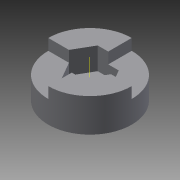
# Autodesk Inventor part: Coil Coupling_1
Saved by Autodesk Inventor 2013 (Build 170138000, 138)
## iProperties
Created: 2013-01-16
Part Number: Coil Coupling_1
Material: Generic
Document SubType Name: Modeling
Designer: Nico
Density: 1 g/cm^3
Author: Nico
Autodesk Inventor part; units mm, degrees
ref_plane "YZ Plane" through (0, 0, 0) normal (1, 0, 0) x (0, 1, 0)
ref_plane "XZ Plane" through (0, 0, 0) normal (0, 1, 0) x (-1, 0, 0)
ref_plane "XY Plane" through (0, 0, 0) normal (0, 0, 1) x (1, 0, 0)
sketch "Sketch1" plane through (0, 0, 0) normal (0, 0, 1) x (1, 0, 0)
  circle A0 centre (0, 0) radius 15
  dimension "d0" = 30
  constraints: 1 centre point, 1 coincident
  measures "d0" diameter of A0
extrude "Extrusion1" add sketch "Sketch1" along normal blind 8
sketch "Sketch2" plane through (0, 0, 8) normal (0, 0, 1) x (1, 0, 0)
  circle A0 centre (0, 0) radius 15 projected
  line L0 (-3.7816, 6.55) -> (0, 6.55)
  line L1 (3.7816, 6.55) -> (7.5633, 0)
  line L2 (7.5633, 0) -> (3.7816, -6.55)
  line L3 (3.7816, -6.55) -> (-3.7816, -6.55)
  line L4 (-3.7816, -6.55) -> (-7.5633, 0)
  line L5 (-7.5633, 0) -> (-3.7816, 6.55)
  line L6 (0, -15) -> (0, -6.55)
  line L7 (-15, 0) -> (-7.5633, 0)
  line L8 (0, 6.55) -> (0, 15)
  line L9 (7.5633, 0) -> (15, 0)
  line L10 (0, 6.55) -> (3.7816, 6.55)
  dimension "d4" = 13.1
  constraints: 22 end point, 6 perpendicular, 4 point on circle, 1 coincident, 1 midpoint, 13 other
  measures "d4" distance between parallel lines of L3 L0
extrude "Extrusion2" add sketch "Sketch2" along normal blind 4 contours A0 L6 L3 L2 L9 | L8 L0 L5 L7 A0
sketch "Sketch3" plane through (0, 0, 8) normal (0, 0, 1) x (1, 0, 0)
  arc A0 (-15, 0) -> (0, -15) centre (0, 0) ccw projected
  line L0 (-3.7816, 6.55) -> (3.7816, 6.55)
  line L1 (3.7816, 6.55) -> (7.5633, 0)
  line L2 (7.5633, 0) -> (3.7816, -6.55)
  line L3 (3.7816, -6.55) -> (-3.7816, -6.55)
  line L4 (-3.7816, -6.55) -> (-7.5633, 0)
  line L5 (-7.5633, 0) -> (-3.7816, 6.55)
  constraints: 12 end point, 1 coincident, 13 other
extrude "Extrusion3" cut sketch "Sketch3" against normal blind 4
sketch "Sketch4" plane through (0, 0, 4) normal (0, 0, 1) x (1, 0, 0)
  circle A0 centre (0, 0) radius 3.9
  dimension "d10" = 7.8
  constraints: 1 centre point, 1 coincident
  measures "d10" diameter of A0
extrude "Extrusion4" cut sketch "Sketch4" against normal blind 10
body "Solid1"
